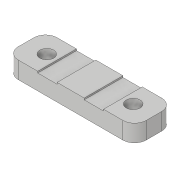
# Autodesk Inventor part: 8 peristaltic pump clamp 0.4mm
Saved by Autodesk Inventor 2020 (Build 240168000, 168)
## iProperties
Created: 2018-08-21
Part Number: 8 peristaltic pump clamp 0.4mm
Material: Generic
Document SubType Name: Modeling
Designer: mrbeh
Density: 1 g/cm^3
Appearance: Default
Author: mrbeh
Autodesk Inventor part; units mm, degrees
ref_plane "YZ Plane" through (0, 0, 0) normal (1, 0, 0) x (0, 1, 0)
ref_plane "XZ Plane" through (0, 0, 0) normal (0, 1, 0) x (-1, 0, 0)
sketch "Sketch1" plane through (0, 0, 0) normal (0, 1, 0) x (-1, 0, 0)
  line L0 (0, 0) -> (33, 0)
  line L1 (33, 0) -> (33, -10)
  line L2 (33, -10) -> (0, -10)
  line L3 (0, -10) -> (0, 0)
  dimension "d0" = 33
  dimension "d1" = 10
  constraints: 8 end point, 2 parallel, 1 horizontal, 1 perpendicular
  measures "d0" distance of L1.end L2.end
  measures "d1" distance of L0.end L1.end
extrude "Extrusion1" add sketch "Sketch1" along normal blind 4
sketch "Sketch2" plane through (0, 4, 0) normal (0, 1, 0) x (1, 0, 0)
  circle A0 centre (-5.343, 5) radius 1.8
  point P0 (0, 0)
  dimension "d9" = 3.6
  constraints: 1 centre point
  measures "d9" diameter of A0
extrude "Extrusion2" cut sketch "Sketch2" against normal blind 4
ref_plane "Work Plane1" through (-16.5, 0, 0) normal (1, 0, 0) x (0, 0, -1)
mirror "Mirror1" about plane through (-16.5, 0, 0) normal (1, 0, 0) of "Extrusion2"
fillet "Fillet1" radius 3 4 edges at (-33, 2, 0) (-33, 2, -10) (0, 2, 0) (0, 2, -10)
sketch "Sketch3" plane through (0, 4, 0) normal (0, 1, 0) x (1, 0, 0)
  line L0 (-30, 0) -> (-3, 0) projected
  line L1 (-30, 10) -> (-3, 10) projected
  line L2 (-20, 0) -> (-13, 0)
  line L3 (-13, 0) -> (-13, 10)
  line L4 (-13, 10) -> (-20, 10)
  line L5 (-20, 10) -> (-20, 0)
  point P0 (0, 0)
  dimension "d10" = 7
  dimension "d11" = 10
  constraints: 8 end point, 2 parallel, 1 horizontal, 1 perpendicular, 1 point on line
  measures "d10" distance of L4.end L3.end
  measures "d11" distance of L3.end L2.end
extrude "Extrusion3" add sketch "Sketch3" along normal blind 0.4
sketch "Sketch4" plane through (0, 4, 0) normal (0, 1, 0) x (1, 0, 0)
  line L0 (-3, 0) -> (-8, 0)
  line L1 (-8, 0) -> (-8, 10)
  line L2 (-8, 10) -> (-3, 10)
  line L3 (0, 7) -> (0, 3)
  arc A0 (-3, 0) -> (0, 3) centre (-3, 3) ccw
  arc A1 (0, 7) -> (-3, 10) centre (-3, 7) ccw
  circle A2 centre (-5.343, 5) radius 1.8 projected
  circle A3 centre (-5.343, 5) radius 1.8
  point P0 (0, 0)
  point P1 (0, 10)
  dimension "d14" = 8
  dimension "d15" = 10
  dimension "d16" = 3
  constraints: 8 end point, 4 point on circle, 4 point on line, 4 tangent, 3 centre point, 2 parallel, 1 coincident, 1 equal radius, 1 horizontal, 1 perpendicular
  measures "d14" distance of L1.end point (0, 10)
  measures "d15" distance of L0.end L1.end
  measures "d16" radius of A0
extrude "Extrusion4" add sketch "Sketch4" along normal blind 0.4
mirror "Mirror2" about plane through (-16.5, 0, 0) normal (1, 0, 0) of "Extrusion4"
sketch "Sketch5" plane through (0, 0, 0) normal (0, -1, 0) x (1, 0, 0)
  line L0 (-24.4942, -3.2042) -> (-8.1968, -3.2042) construction
  line L1 (-8.1968, -3.2042) -> (-8.1968, -6.8489) construction
  line L2 (-8.1968, -6.8489) -> (-24.4942, -6.8489) construction
  line L3 (-24.4942, -6.8489) -> (-24.4942, -3.2042) construction
  spline S0 degree 2 poles (-22.0607, -5.0252) (-22.0607, -5.9668) (-22.6081, -6.8489) (-23.1782, -6.8489) knots 0 0 0 1 2 2 2
  spline S1 degree 2 poles (-23.1782, -6.8489) (-23.7568, -6.8489) (-24.2985, -5.9498) (-24.2985, -5.028) knots 0 0 0 1 2 2 2
  spline S2 degree 2 poles (-24.2985, -5.028) (-24.2985, -4.0807) (-23.7511, -3.2042) (-23.1782, -3.2042) knots 0 0 0 1 2 2 2
  spline S3 degree 2 poles (-23.1782, -3.2042) (-22.6024, -3.2042) (-22.0607, -4.1119) (-22.0607, -5.0252) knots 0 0 0 1 2 2 2
  spline S4 degree 2 poles (-22.662, -6.0916) (-22.5939, -5.9186) (-22.5372, -5.3854) (-22.5372, -5.0252) knots 0 0 0 1 2 2 2
  spline S5 degree 2 poles (-22.5372, -5.0252) (-22.5372, -4.6649) (-22.5939, -4.1346) (-22.6648, -3.9559) knots 0 0 0 1 2 2 2
  spline S6 degree 2 poles (-22.6648, -3.9559) (-22.7357, -3.7772) (-22.9825, -3.5928) (-23.1782, -3.5928) knots 0 0 0 1 2 2 2
  spline S7 degree 2 poles (-23.1782, -3.5928) (-23.3739, -3.5928) (-23.6263, -3.7772) (-23.7, -3.9615) knots 0 0 0 1 2 2 2
  spline S8 degree 2 poles (-23.7, -3.9615) (-23.7709, -4.1402) (-23.822, -4.6848) (-23.822, -5.028) knots 0 0 0 1 2 2 2
  spline S9 degree 2 poles (-23.822, -5.028) (-23.822, -5.3967) (-23.7766, -5.8902) (-23.7029, -6.0831) knots 0 0 0 1 2 2 2
  spline S10 degree 2 poles (-23.7029, -6.0831) (-23.6348, -6.2646) (-23.3824, -6.4603) (-23.1782, -6.4603) knots 0 0 0 1 2 2 2
  spline S11 degree 2 poles (-23.1782, -6.4603) (-22.9853, -6.4603) (-22.7329, -6.276) (-22.662, -6.0916) knots 0 0 0 1 2 2 2
  line L4 (-20.8609, -6.7752) -> (-21.4225, -6.7752)
  line L5 (-21.4225, -6.7752) -> (-21.4225, -6.1058)
  line L6 (-21.4225, -6.1058) -> (-20.8609, -6.1058)
  line L7 (-20.8609, -6.1058) -> (-20.8609, -6.7752)
  line L8 (-17.9026, -5.5726) -> (-18.3196, -5.5726)
  line L9 (-18.3196, -5.5726) -> (-18.3196, -6.7752)
  line L10 (-18.3196, -6.7752) -> (-18.7705, -6.7752)
  line L11 (-18.7705, -6.7752) -> (-18.7705, -5.5726)
  line L12 (-18.7705, -5.5726) -> (-20.3163, -5.5726)
  line L13 (-20.3163, -5.5726) -> (-20.3163, -5.079)
  line L14 (-20.3163, -5.079) -> (-18.7507, -3.2752)
  line L15 (-18.7507, -3.2752) -> (-18.3196, -3.2752)
  line L16 (-18.3196, -3.2752) -> (-18.3196, -5.1953)
  line L17 (-18.3196, -5.1953) -> (-17.9026, -5.1953)
  line L18 (-17.9026, -5.1953) -> (-17.9026, -5.5726)
  line L19 (-18.7705, -5.1953) -> (-18.7705, -3.8282)
  line L20 (-18.7705, -3.8282) -> (-19.9476, -5.1953)
  line L21 (-19.9476, -5.1953) -> (-18.7705, -5.1953)
  line L22 (-12.9816, -6.7752) -> (-12.9816, -5.2549)
  spline S12 degree 2 poles (-12.9816, -5.2549) (-12.9816, -5.0734) (-13.01, -4.7642) (-13.0554, -4.6791) knots 0 0 0 1 2 2 2
  spline S13 degree 2 poles (-13.0554, -4.6791) (-13.1008, -4.5855) (-13.2738, -4.4948) (-13.4241, -4.4948) knots 0 0 0 1 2 2 2
  spline S14 degree 2 poles (-13.4241, -4.4948) (-13.5603, -4.4948) (-13.8722, -4.6621) (-14.0368, -4.8209) knots 0 0 0 1 2 2 2
  spline S15 degree 2 poles (-14.0368, -4.8209) (-14.0339, -4.8606) (-14.0282, -4.9713) (-14.0282, -5.045) knots 0 0 0 1 2 2 2
  line L23 (-14.0282, -5.045) -> (-14.0282, -6.7752)
  line L24 (-14.0282, -6.7752) -> (-14.4707, -6.7752)
  line L25 (-14.4707, -6.7752) -> (-14.4707, -5.2549)
  spline S16 degree 2 poles (-14.4707, -5.2549) (-14.4707, -5.0734) (-14.4991, -4.7642) (-14.5444, -4.6791) knots 0 0 0 1 2 2 2
  spline S17 degree 2 poles (-14.5444, -4.6791) (-14.5898, -4.5855) (-14.7628, -4.4948) (-14.9132, -4.4948) knots 0 0 0 1 2 2 2
  spline S18 degree 2 poles (-14.9132, -4.4948) (-15.055, -4.4948) (-15.3698, -4.6735) (-15.5173, -4.8124) knots 0 0 0 1 2 2 2
  line L26 (-15.5173, -4.8124) -> (-15.5173, -6.7752)
  line L27 (-15.5173, -6.7752) -> (-15.9598, -6.7752)
  line L28 (-15.9598, -6.7752) -> (-15.9598, -4.1487)
  line L29 (-15.9598, -4.1487) -> (-15.5173, -4.1487)
  line L30 (-15.5173, -4.1487) -> (-15.5173, -4.438)
  spline S19 degree 2 poles (-15.5173, -4.438) (-15.3443, -4.265) (-15.0039, -4.075) (-14.7997, -4.075) knots 0 0 0 1 2 2 2
  spline S20 degree 2 poles (-14.7997, -4.075) (-14.5671, -4.075) (-14.2069, -4.2877) (-14.1133, -4.5288) knots 0 0 0 1 2 2 2
  spline S21 degree 2 poles (-14.1133, -4.5288) (-13.912, -4.3047) (-13.5319, -4.075) (-13.3107, -4.075) knots 0 0 0 1 2 2 2
  spline S22 degree 2 poles (-13.3107, -4.075) (-13.1405, -4.075) (-12.8625, -4.1799) (-12.7604, -4.2991) knots 0 0 0 1 2 2 2
  spline S23 degree 2 poles (-12.7604, -4.2991) (-12.6555, -4.4182) (-12.5392, -4.7756) (-12.5392, -5.045) knots 0 0 0 1 2 2 2
  line L31 (-12.5392, -5.045) -> (-12.5392, -6.7752)
  line L32 (-12.5392, -6.7752) -> (-12.9816, -6.7752)
  line L33 (-8.9399, -6.7752) -> (-8.9399, -5.2549)
  spline S24 degree 2 poles (-8.9399, -5.2549) (-8.9399, -5.0734) (-8.9683, -4.7642) (-9.0137, -4.6791) knots 0 0 0 1 2 2 2
  spline S25 degree 2 poles (-9.0137, -4.6791) (-9.059, -4.5855) (-9.2321, -4.4948) (-9.3824, -4.4948) knots 0 0 0 1 2 2 2
  spline S26 degree 2 poles (-9.3824, -4.4948) (-9.5185, -4.4948) (-9.8305, -4.6621) (-9.995, -4.8209) knots 0 0 0 1 2 2 2
  spline S27 degree 2 poles (-9.995, -4.8209) (-9.9922, -4.8606) (-9.9865, -4.9713) (-9.9865, -5.045) knots 0 0 0 1 2 2 2
  line L34 (-9.9865, -5.045) -> (-9.9865, -6.7752)
  line L35 (-9.9865, -6.7752) -> (-10.429, -6.7752)
  line L36 (-10.429, -6.7752) -> (-10.429, -5.2549)
  spline S28 degree 2 poles (-10.429, -5.2549) (-10.429, -5.0734) (-10.4573, -4.7642) (-10.5027, -4.6791) knots 0 0 0 1 2 2 2
  spline S29 degree 2 poles (-10.5027, -4.6791) (-10.5481, -4.5855) (-10.7211, -4.4948) (-10.8714, -4.4948) knots 0 0 0 1 2 2 2
  spline S30 degree 2 poles (-10.8714, -4.4948) (-11.0133, -4.4948) (-11.3281, -4.6735) (-11.4756, -4.8124) knots 0 0 0 1 2 2 2
  line L37 (-11.4756, -4.8124) -> (-11.4756, -6.7752)
  line L38 (-11.4756, -6.7752) -> (-11.918, -6.7752)
  line L39 (-11.918, -6.7752) -> (-11.918, -4.1487)
  line L40 (-11.918, -4.1487) -> (-11.4756, -4.1487)
  line L41 (-11.4756, -4.1487) -> (-11.4756, -4.438)
  spline S31 degree 2 poles (-11.4756, -4.438) (-11.3026, -4.265) (-10.9622, -4.075) (-10.758, -4.075) knots 0 0 0 1 2 2 2
  spline S32 degree 2 poles (-10.758, -4.075) (-10.5254, -4.075) (-10.1652, -4.2877) (-10.0716, -4.5288) knots 0 0 0 1 2 2 2
  spline S33 degree 2 poles (-10.0716, -4.5288) (-9.8702, -4.3047) (-9.4902, -4.075) (-9.2689, -4.075) knots 0 0 0 1 2 2 2
  spline S34 degree 2 poles (-9.2689, -4.075) (-9.0987, -4.075) (-8.8208, -4.1799) (-8.7187, -4.2991) knots 0 0 0 1 2 2 2
  spline S35 degree 2 poles (-8.7187, -4.2991) (-8.6137, -4.4182) (-8.4974, -4.7756) (-8.4974, -5.045) knots 0 0 0 1 2 2 2
  line L42 (-8.4974, -5.045) -> (-8.4974, -6.7752)
  line L43 (-8.4974, -6.7752) -> (-8.9399, -6.7752)
  point P0 (0, 0)
  constraints: 2 other
extrude "Extrusion5" add sketch "Sketch5" along normal blind 0.5
body "Solid1"
